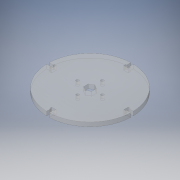
# Autodesk Inventor part: PlexiHalter1
Saved by Autodesk Inventor 2016 (Build 200138000, 138)
## iProperties
Created: 2018-05-15
Part Number: PlexiHalter1
Material: Polycarbonate, Clear
Document SubType Name: Modeling
Designer: Phil Erle
Density: 1.2 g/cm^3
Appearance: Polycarbonate - Clear
Author: Phil Erle
Autodesk Inventor part; units mm, degrees
ref_plane "YZ Plane" through (0, 0, 0) normal (1, 0, 0) x (0, 1, 0)
ref_plane "XZ Plane" through (0, 0, 0) normal (0, 1, 0) x (-1, 0, 0)
ref_plane "XY Plane" through (0, 0, 0) normal (0, 0, 1) x (1, 0, 0)
sketch "Sketch1" plane through (0, 0, 0) normal (0, 0, 1) x (1, 0, 0)
  circle A0 centre (0, 0) radius 51
  dimension "d0" = 102
  constraints: 1 centre point, 1 coincident
  measures "d0" diameter of A0
extrude "Extrusion1" add sketch "Sketch1" along normal blind 5
sketch "Sketch2" plane through (0, 0, 0) normal (0, 0, -1) x (-1, 0, 0)
  line L0 (0, 5.7735) -> (5, 2.8868)
  line L1 (5, 2.8868) -> (5, -2.8868)
  line L2 (5, -2.8868) -> (0, -5.7735)
  line L3 (0, -5.7735) -> (-5, -2.8868)
  line L4 (-5, -2.8868) -> (-5, 2.8868)
  line L5 (-5, 2.8868) -> (0, 5.7735)
  point P0 (0, 0)
  point P1 (0, 0)
  dimension "d3" = 10
  constraints: 12 end point, 1 coincident, 1 vertical alignment, 13 other
  measures "d3" distance between parallel lines of L4 L1
extrude "Extrusion2" cut sketch "Sketch2" against normal blind 5
sketch "Sketch3" plane through (0, 0, 0) normal (0, 0, -1) x (-1, 0, 0)
  circle A0 centre (0, 0) radius 15 construction
  point P0 (0, 15)
  point P1 (15, 0)
  point P2 (0, -15)
  point P3 (-15, 0)
  dimension "d6" = 30
  constraints: 4 point on circle, 2 horizontal alignment, 2 vertical alignment, 1 centre point, 1 coincident
  measures "d6" diameter of A0
hole "Hole1" at (0, 15, 0) at (-15, 0, 0) at (0, -15, 0) at (15, 0, 0) direction (0, 0, 1) diameter 3.4 depth 8 tip angle 118 clearance for "Countersunk Flat Head Screw DIN EN ISO 2009" size "M3" standard "DIN"
sketch "Sketch4" plane through (0, 0, 0) normal (0, 0, -1) x (-1, 0, 0)
  line L0 (-1.6, 51) -> (1.6, 51)
  line L1 (1.6, 51) -> (1.6, 46)
  line L2 (1.6, 46) -> (-2.75, 46)
  line L3 (-2.75, 46) -> (-2.75, 43.6)
  line L4 (-2.75, 43.6) -> (2.75, 43.6)
  line L5 (2.75, 43.6) -> (2.75, 46)
  line L6 (2.75, 46) -> (-1.6, 46)
  line L7 (-1.6, 46) -> (-1.6, 51)
  line L8 (-51, -1.6) -> (-51, 1.6)
  line L9 (-51, 1.6) -> (-46, 1.6)
  line L10 (-46, 1.6) -> (-46, -2.75)
  line L11 (-46, -2.75) -> (-43.6, -2.75)
  line L12 (-43.6, -2.75) -> (-43.6, 2.75)
  line L13 (-43.6, 2.75) -> (-46, 2.75)
  line L14 (-46, 2.75) -> (-46, -1.6)
  line L15 (-46, -1.6) -> (-51, -1.6)
  line L16 (1.6, -51) -> (-1.6, -51)
  line L17 (-1.6, -51) -> (-1.6, -46)
  line L18 (-1.6, -46) -> (2.75, -46)
  line L19 (2.75, -46) -> (2.75, -43.6)
  line L20 (2.75, -43.6) -> (-2.75, -43.6)
  line L21 (-2.75, -43.6) -> (-2.75, -46)
  line L22 (-2.75, -46) -> (1.6, -46)
  line L23 (1.6, -46) -> (1.6, -51)
  line L24 (51, 1.6) -> (51, -1.6)
  line L25 (51, -1.6) -> (46, -1.6)
  line L26 (46, -1.6) -> (46, 2.75)
  line L27 (46, 2.75) -> (43.6, 2.75)
  line L28 (43.6, 2.75) -> (43.6, -2.75)
  line L29 (43.6, -2.75) -> (46, -2.75)
  line L30 (46, -2.75) -> (46, 1.6)
  line L31 (46, 1.6) -> (51, 1.6)
  point P0 (0, 0)
  point P1 (0, 43.6)
  point P2 (0, 51)
  point P3 (-51, 0)
  point P4 (-43.6, 0)
  point P5 (0, -51)
  point P6 (0, -43.6)
  point P7 (51, 0)
  point P8 (43.6, 0)
  dimension "d14" = 5
  dimension "d15" = 2.4
  dimension "d16" = 5.5
  dimension "d17" = 3.2
  dimension "d18" = 51
  dimension "d21" = 360
  constraints: 64 end point, 8 point on line, 6 perpendicular, 2 midpoint, 2 vertical alignment, 1 horizontal, 73 other
  measures "d14" distance of L6.end L0.start
  measures "d15" distance of L4.end L5.end
  measures "d16" distance of L3.end L4.end
  measures "d17" distance of L0.start L0.end
  measures "d18" distance of point (0, 0) point (0, 51)
extrude "Extrusion3" cut sketch "Sketch4" against normal through all
body "Solid1"
